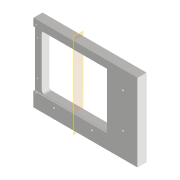
# Autodesk Inventor part: 30_XYTabel_Aliexpress_xslide
Saved by Autodesk Inventor 2022 (Build 260153000, 153)
## iProperties
Created: 2021-12-30
Part Number: 30_XYTabel_Aliexpress_xslide
Material: Generisch
Document SubType Name: Modeling
Designer: diederichbenedict
Density: 1 g/cm^3
Appearance: Vorgabe
Author: diederichbenedict
Autodesk Inventor part; units mm, degrees
ref_plane "YZ Plane" through (0, 0, 0) normal (1, 0, 0) x (0, 1, 0)
ref_plane "XZ Plane" through (0, 0, 0) normal (0, 1, 0) x (-1, 0, 0)
ref_plane "XY Plane" through (0, 0, 0) normal (0, 0, 1) x (1, 0, 0)
sketch "Skizze1" plane through (0, 0, 0) normal (0, 0, 1) x (1, 0, 0)
  line L0 (52.68, 47.5) -> (-52.68, 47.5)
  line L1 (-57.68, 42.5) -> (-57.68, -42.5)
  line L2 (-52.68, -47.5) -> (52.68, -47.5)
  line L3 (57.68, -42.5) -> (57.68, 42.5)
  line L4 (57.68, 47.5) -> (-57.68, -47.5) construction
  line L5 (-57.68, 47.5) -> (57.68, -47.5) construction
  arc A0 (-52.68, 47.5) -> (-57.68, 42.5) centre (-52.68, 42.5) ccw
  arc A1 (57.68, 42.5) -> (52.68, 47.5) centre (52.68, 42.5) ccw
  arc A2 (52.68, -47.5) -> (57.68, -42.5) centre (52.68, -42.5) ccw
  arc A3 (-57.68, -42.5) -> (-52.68, -47.5) centre (-52.68, -42.5) ccw
  line L6 (110.38, -72.86) -> (-69.3, -72.86)
  line L7 (-69.3, -72.86) -> (-69.3, 61.32)
  line L8 (-69.3, 61.32) -> (110.38, 61.32)
  line L9 (110.38, 61.32) -> (110.38, -72.86)
  point P0 (0, 0)
  dimension "d0" = 115.36
  dimension "d1" = 95
  dimension "d2" = 5
  dimension "d3" = 52.7
  dimension "d4" = 25.36
  dimension "d5" = 11.62
  dimension "d6" = 13.82
  constraints: 20 end point, 8 point on circle, 8 point on line, 8 tangent, 4 centre point, 4 parallel, 3 equal radius, 2 horizontal, 2 midpoint, 2 perpendicular
  measures "d0" distance of L5.end L4.end
  measures "d1" distance between parallel lines of L2 L0
  measures "d2" radius of A0
  measures "d3" distance between parallel lines of L9 L3
  measures "d4" distance between parallel lines of L6 L2
  measures "d5" distance between parallel lines of L7 L1
  measures "d6" distance between parallel lines of L8 L0
extrude "Extrusion1" add sketch "Skizze1" along normal blind 12.82
sketch "Skizze2" plane through (0, 0, 12.82) normal (0, 0, 1) x (1, 0, 0)
  line L0 (110.38, 61.32) -> (-69.3, 61.32) projected
  line L1 (-69.3, 61.32) -> (-69.3, -72.86) projected
  line L2 (-69.3, -72.86) -> (110.38, -72.86) projected
  line L3 (110.38, -72.86) -> (110.38, 61.32) projected
  arc A0 (57.68, 42.5) -> (52.68, 47.5) centre (52.68, 42.5) ccw projected
  line L4 (57.68, 42.5) -> (57.68, -42.5) projected
  arc A1 (52.68, -47.5) -> (57.68, -42.5) centre (52.68, -42.5) ccw projected
  line L5 (52.68, -47.5) -> (-52.68, -47.5) projected
  arc A2 (-57.68, -42.5) -> (-52.68, -47.5) centre (-52.68, -42.5) ccw projected
  line L6 (-57.68, -42.5) -> (-57.68, 42.5) projected
  arc A3 (-52.68, 47.5) -> (-57.68, 42.5) centre (-52.68, 42.5) ccw projected
  line L7 (-52.68, 47.5) -> (52.68, 47.5) projected
  line L8 (-74.2294, 48.44) -> (57.68, 48.44)
  line L9 (57.68, 48.44) -> (57.68, -47.9)
  line L10 (57.68, -47.9) -> (-74.2294, -47.9)
  line L11 (-74.2294, -47.9) -> (-74.2294, 48.44)
  point P0 (0, 0)
  point P1 (-69.3, 48.44)
  point P2 (-69.3, -47.9)
  dimension "d9" = 12.88
  dimension "d10" = 0.4
  constraints: 8 end point, 2 parallel, 1 horizontal, 1 perpendicular
  measures "d9" distance between parallel lines of L8 L0
  measures "d10" distance between parallel lines of L5 L10
extrude "Extrusion2" add sketch "Skizze2" along normal blind 2.77 contours L3 L2 L1 L10 L9 L4 L8 L0
sketch "Skizze3" plane through (0, 0, 15.59) normal (0, 0, 1) x (1, 0, 0)
  line L0 (-69.3, 61.32) -> (-69.3, 48.44) projected
  line L1 (-69.3, 48.44) -> (57.68, 48.44) projected
  line L2 (57.68, 48.44) -> (57.68, -47.9) projected
  line L3 (57.68, -47.9) -> (-69.3, -47.9) projected
  line L4 (-69.3, -47.9) -> (-69.3, -72.86) projected
  line L5 (-69.3, -72.86) -> (110.38, -72.86) projected
  line L6 (110.38, -72.86) -> (110.38, 61.32) projected
  line L7 (110.38, 61.32) -> (-69.3, 61.32) projected
  circle A0 centre (-64.8, 52.82) radius 1
  circle A1 centre (-64.8, 32) radius 1
  circle A2 centre (-64.8, -28.6) radius 1
  circle A3 centre (85.38, 29.82) radius 1.5
  circle A4 centre (85.38, -30.68) radius 1.5
  circle A5 centre (32.2, -56.36) radius 1.5
  circle A6 centre (-33.8, -56.36) radius 1.5
  circle A7 centre (-64.8, -49.18) radius 1
  line L8 (-69.3, 48.44) -> (-69.3, -47.9) projected
  point P0 (0, 0)
  dimension "d13" = 2
  dimension "d14" = 2
  dimension "d15" = 2
  dimension "d16" = 3
  dimension "d17" = 3
  dimension "d18" = 3
  dimension "d19" = 3
  dimension "d20" = 2
  dimension "d21" = 8.5
  dimension "d22" = 4.5
  dimension "d23" = 4.5
  dimension "d24" = 4.5
  dimension "d25" = 4.5
  dimension "d26" = 20.82
  dimension "d27" = 81.42
  dimension "d28" = 102
  dimension "d29" = 16.5
  dimension "d30" = 16.5
  dimension "d31" = 66
  dimension "d32" = 35.5
  dimension "d33" = 25
  dimension "d34" = 25
  dimension "d35" = 31.5
  dimension "d36" = 60.5
  constraints: 8 centre point
  measures "d13" diameter of A0
  measures "d14" diameter of A1
  measures "d15" diameter of A2
  measures "d16" diameter of A3
  measures "d17" diameter of A4
  measures "d18" diameter of A5
  measures "d19" diameter of A6
  measures "d20" diameter of A7
  measures "d21" distance from line of A0.centre L7
  measures "d22" distance from line of L0 A0.centre
  measures "d23" distance from line of L8 A1.centre
  measures "d24" distance from line of L8 A2.centre
  measures "d25" distance from line of L4 A7.centre
  measures "d26" distance of A1.centre A0.centre
  measures "d27" distance of A2.centre A0.centre
  measures "d28" distance of A7.centre A0.centre
  measures "d29" distance from line of A6.centre L5
  measures "d30" distance from line of A5.centre L5
  measures "d31" distance of A5.centre A6.centre
  measures "d32" distance from line of L4 A6.centre
  measures "d33" distance from line of A3.centre L6
  measures "d34" distance from line of A4.centre L6
  measures "d35" distance from line of A3.centre L7
  measures "d36" distance of A3.centre A4.centre
extrude "Extrusion3" cut sketch "Skizze3" against normal through all contours A0 | A1 | A2 | A3 | A4 | A5 | A6 | A7
sketch "Skizze4" plane through (0, 0, 0) normal (0, 0, -1) x (-1, 0, 0)
  circle A0 centre (-85.38, -30.68) radius 1.5 projected
  circle A1 centre (64.8, -28.6) radius 1 projected
  circle A2 centre (64.8, -49.18) radius 1 projected
  circle A3 centre (-85.38, 29.82) radius 1.5 projected
  circle A4 centre (-32.2, -56.36) radius 1.5 projected
  circle A5 centre (64.8, 32) radius 1 projected
  circle A6 centre (33.8, -56.36) radius 1.5 projected
  circle A7 centre (64.8, 52.82) radius 1 projected
  line L0 (-110.38, 61.32) -> (69.3, 61.32) projected
  line L1 (-110.38, -72.86) -> (-110.38, 61.32) projected
  line L2 (69.3, -72.86) -> (-110.38, -72.86) projected
  line L3 (69.3, 61.32) -> (69.3, -72.86) projected
  arc A8 (-52.68, 47.5) -> (-57.68, 42.5) centre (-52.68, 42.5) ccw projected
  line L4 (52.68, 47.5) -> (-52.68, 47.5) projected
  arc A9 (57.68, 42.5) -> (52.68, 47.5) centre (52.68, 42.5) ccw projected
  line L5 (57.68, -42.5) -> (57.68, 42.5) projected
  arc A10 (52.68, -47.5) -> (57.68, -42.5) centre (52.68, -42.5) ccw projected
  line L6 (-52.68, -47.5) -> (52.68, -47.5) projected
  arc A11 (-57.68, -42.5) -> (-52.68, -47.5) centre (-52.68, -42.5) ccw projected
  line L7 (-57.68, 42.5) -> (-57.68, -42.5) projected
  circle A12 centre (15.46, 44) radius 1
  circle A13 centre (-20.54, 44) radius 1
  point P0 (0, 0)
  dimension "d39" = 2
  dimension "d40" = 2
  dimension "d41" = 3.5
  dimension "d42" = 3.5
  dimension "d43" = 36
  constraints: 2 centre point
  measures "d39" diameter of A12
  measures "d40" diameter of A13
  measures "d41" distance from line of A12.centre L4
  measures "d42" distance from line of A13.centre L4
  measures "d43" distance of A13.centre A12.centre
extrude "Extrusion4" add sketch "Skizze4" against normal blind 10 contours A12 | A13
ref_plane "Arbeitsebene1" through (0, -42.5, 0) normal (1, 0, 0) x (0, 0, -1)
